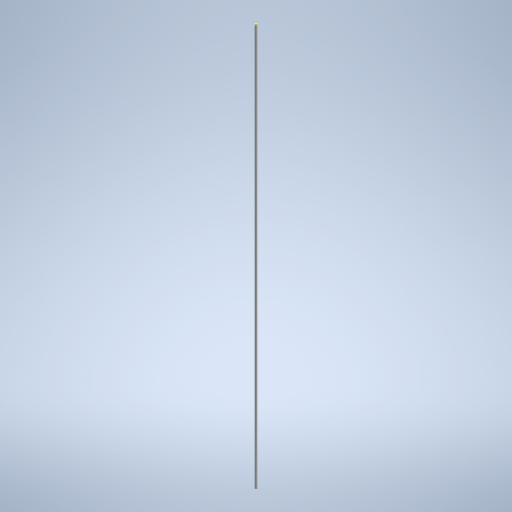
# Autodesk Inventor part: tige filetée
Saved by Autodesk Inventor 2023 (Build 270158000, 158)
## iProperties
Created: 2023-04-12
Part Number: tige filetée
Material: Générique
Document SubType Name: Modeling
Designer: Julia
Density: 1 g/cm^3
Appearance: Par défaut
Author: Julia
Autodesk Inventor part; units mm, degrees
ref_plane "YZ Plane" through (0, 0, 0) normal (1, 0, 0) x (0, 1, 0)
ref_plane "XZ Plane" through (0, 0, 0) normal (0, 1, 0) x (-1, 0, 0)
ref_plane "XY Plane" through (0, 0, 0) normal (0, 0, 1) x (1, 0, 0)
sketch "Esquisse3" plane through (0, 0, 0) normal (0, 1, 0) x (-1, 0, 0)
  circle A0 centre (0, 0) radius 3
  dimension "d3" = 6
  constraints: 1 centre point, 1 coincident
  measures "d3" diameter of A0
extrude "Extrusion2" add sketch "Esquisse3" along normal mid plane 1300
sketch "Esquisse4" plane through (0, 650, 0) normal (0, 1, 0) x (1, 0, 0)
  point P0 (0, 0)
thread "Filetage1" size "1/4-20 UNC" class "1A" standard "ANSI Unified Screw Threads" full length
